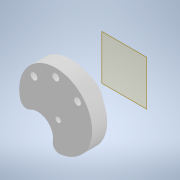
# Autodesk Inventor part: main_wheel_fixator_mirror
Saved by Autodesk Inventor 2022 (Build 260153000, 153)
## iProperties
Created: 2024-09-10
Part Number: main_wheel_fixator_mirror
Material: Типовые
Document SubType Name: Modeling
Designer: Andrey
Density: 1 g/cm^3
Appearance: По умолчанию
Author: Andrey
Autodesk Inventor part; units mm, degrees
ref_plane "YZ Plane" through (0, 0, 0) normal (1, 0, 0) x (0, 1, 0)
ref_plane "XZ Plane" through (0, 0, 0) normal (0, 1, 0) x (-1, 0, 0)
ref_plane "XY Plane" through (0, 0, 0) normal (0, 0, 1) x (1, 0, 0)
ref_plane "РабПлоскость1" through (-130.0323, -33.3842, -9.2947) normal (0, 0, 1) x (1, 0, 0)
sketch "Эскиз1" plane through (0, 0, 0) normal (0, 0, 1) x (1, 0, 0)
  circle A0 centre (0, 0) radius 22.5
  dimension "d0" = 45
  constraints: 1 centre point, 1 coincident
  measures "d0" diameter of A0
extrude "Выдавливание1" add sketch "Эскиз1" against normal up to surface (9.2947 mm away)
sketch "Эскиз2" plane through (0, 0, 0) normal (0, 0, 1) x (1, 0, 0)
  arc A0 (-12.5314, -17.4431) -> (-12.5619, -14.5867) centre (-11.1467, -16) ccw projected
  circle A1 centre (-11.1467, -16) radius 6.5
  circle A2 centre (-11.1467, -16) radius 9.5
  point P0 (0, 0)
  dimension "d3" = 13
  dimension "d4" = 3
  constraints: 2 centre point, 1 coincident
  measures "d3" diameter of A1
  measures "d4" radial gap between concentric circles of A1 A2
extrude "Выдавливание2" cut sketch "Эскиз2" against normal blind 10 contours A1 | A2
fillet "Сопряжение1" radius 4 2 edges at (-3.9122, -22.1573, -4.6474) (-19.4292, -11.347, -4.6474)
sketch "Эскиз3" plane through (0, 0, 0) normal (0, 0, 1) x (1, 0, 0)
  circle A0 centre (0, 0) radius 12.6
  line L0 (0, 0) -> (0, -4)
  line L1 (0, -4) -> (-3.4641, -2)
  line L2 (-3.4641, -2) -> (-3.4641, 2)
  line L3 (-3.4641, 2) -> (0, 4)
  line L4 (0, 4) -> (3.4641, 2)
  line L5 (3.4641, 2) -> (3.4641, -2)
  line L6 (3.4641, -2) -> (0, -4)
  line L7 (-3.9641, -2.2887) -> (0, -4.5774)
  line L8 (0, -4.5774) -> (3.9641, -2.2887)
  line L9 (3.9641, -2.2887) -> (3.9641, 2.2887)
  line L10 (3.9641, 2.2887) -> (0, 4.5774)
  line L11 (0, 4.5774) -> (-3.9641, 2.2887)
  line L12 (-3.9641, 2.2887) -> (-3.9641, -2.2887)
  arc A1 (-21.8671, -5.2989) -> (-15.9551, -7.8067) centre (-17.9796, -4.3569) ccw projected
  arc A2 (-1.795, -17.6717) -> (-15.9551, -7.8067) centre (-11.1467, -16) ccw projected
  arc A3 (-1.795, -17.6717) -> (2.6059, -22.3486) centre (2.1426, -18.3755) ccw projected
  arc A4 (2.6059, -22.3486) -> (-21.8671, -5.2989) centre (0, 0) ccw projected
  point P0 (-10.7899, -6.5067)
  point P1 (-2.3651, -12.376)
  dimension "d8" = 25.2
  dimension "d9" = 4
  dimension "d10" = 0.5
  constraints: 26 end point, 2 coincident, 1 centre point, 1 vertical, 18 other
  measures "d8" diameter of A0
  measures "d9" distance of L0.start L0.end
  measures "d10" distance between parallel lines of L1 L7
extrude "Выдавливание3" add sketch "Эскиз3" along normal blind 7.8 contours A0 A2 picked at (6.8427, 0)
sketch "Эскиз4" plane through (0, 0, 0) normal (0, 0, 1) x (1, 0, 0)
  arc A0 (-2.3651, -12.376) -> (-10.7899, -6.5067) centre (0, 0) ccw projected
  arc A1 (-1.795, -17.6717) -> (-2.3651, -12.376) centre (-11.1467, -16) ccw projected
  arc A2 (-1.795, -17.6717) -> (2.6059, -22.3486) centre (2.1426, -18.3755) ccw projected
  arc A3 (2.6059, -22.3486) -> (-21.8671, -5.2989) centre (0, 0) ccw projected
  arc A4 (-21.8671, -5.2989) -> (-15.9551, -7.8067) centre (-17.9796, -4.3569) ccw projected
  arc A5 (-10.7899, -6.5067) -> (-15.9551, -7.8067) centre (-11.1467, -16) ccw projected
  circle A6 centre (0, 0) radius 12.6
  circle A7 centre (0, 0) radius 14.6
  point P0 (-1.7671, -14.4927)
  point P1 (-12.9827, -6.6791)
  dimension "d13" = 2
  constraints: 2 centre point, 1 coincident, 1 concentric
  measures "d13" radial gap between concentric circles of A6 A7
extrude "Выдавливание4" add sketch "Эскиз4" along normal blind 1 contours A0 A5 A7 A1
fillet "Сопряжение2" radius 2 4 edges at (-2.3651, -12.376, 4.4) (-1.7671, -14.4927, 0.5) (-10.7899, -6.5067, 4.4) (-12.9827, -6.6791, 0.5)
chamfer "Фаска1" distance 0.5 angle 45 7 edges at (8.3458, 11.9795, 1) (-12.8509, -6.1946, 1) (-11.2228, -6.5003, 1) (-10.3052, -6.5373, 1) (-1.3582, -14.2012, 1) (-2.2091, -12.7799, 1) (-2.5618, -11.932, 1)
sketch "Эскиз5" plane through (0, 0, -9.2947) normal (0, 0, -1) x (-0.8205128, 0.5716281, 0)
  circle A0 centre (-6.9744, -14.6412) radius 1.5
  arc A1 (5.5942, -23.7713) -> (7.8344, -23.1299) centre (6.9744, -24.3588) ccw
  arc A2 (5.5942, -23.7713) -> (5.8702, -23.7046) centre (0, 0) ccw
  spline S0 degree 3 poles (7.0407, -25.2882) (6.986, -25.2268) (6.8766, -25.1041) (6.7176, -24.9155) (6.5628, -24.7236) (6.4128, -24.5278) (6.2678, -24.3283) (6.1284, -24.1248) (6.0175, -23.9518) (5.9319, -23.8114) (5.8908, -23.7402) (5.8702, -23.7046) knots 0 0 0 0 0.125 0.250001 0.375002 0.500002 0.625001 0.75 0.874998 0.937499 1 1 1 1
  arc A3 (7.0407, -25.2882) -> (7.5579, -25.1384) centre (0, 0) ccw
  spline S1 degree 3 poles (7.7014, -23.1745) (7.703, -23.2156) (7.7063, -23.2977) (7.709, -23.4621) (7.7076, -23.6676) (7.6985, -23.9141) (7.6826, -24.1602) (7.6603, -24.4058) (7.632, -24.6508) (7.5984, -24.8952) (7.5714, -25.0573) (7.5579, -25.1384) knots 0 0 0 0 0.062501 0.125002 0.25 0.374999 0.499998 0.624998 0.749999 0.875 1 1 1 1
  arc A4 (7.7014, -23.1745) -> (7.8344, -23.1299) centre (0, 0) ccw
  circle A5 centre (0, -19.5) radius 4.5
  line L0 (-92.3726, 48.2814) -> (-109.8668, 39.9786)
  line L1 (13.2101, -45.7656) -> (-109.8668, 39.9786)
  line L2 (13.2101, -45.7656) -> (14.9372, -26.4783)
  arc A6 (18.1683, -19.9728) -> (14.9372, -26.4783) centre (24.8973, -27.3701) ccw
  arc A7 (18.1683, -19.9728) -> (-19.7633, 18.396) centre (0, 0) ccw
  arc A8 (-26.2813, 17.7001) -> (-19.7633, 18.396) centre (-23.4232, 21.8026) ccw
  line L3 (-26.2813, 17.7001) -> (-36.6493, 24.9232)
  arc A9 (-38.2549, 31.2785) -> (-36.6493, 24.9232) centre (-33.7911, 29.0257) ccw
  arc A10 (-38.2549, 31.2785) -> (-87.3896, 53.5664) centre (-62.359, 43.4437) ccw
  arc A11 (-92.3726, 48.2814) -> (-87.3896, 53.5664) centre (-96.6602, 57.3156) ccw
  circle A12 centre (-4.5825, 16.9412) radius 2.1
  circle A13 centre (10.0321, 14.4) radius 2.1
  circle A14 centre (17.4795, 1.5711) radius 2.1
  circle A15 centre (10.0321, 14.4) radius 3.5
  circle A16 centre (-4.5825, 16.9412) radius 3.5
  circle A17 centre (17.4795, 1.5711) radius 3.5
  circle A18 centre (-52.3269, 57.8437) radius 3.5
  circle A19 centre (-44.8794, 45.0149) radius 3.5
  circle A20 centre (-66.9415, 60.3849) radius 3.5
  circle A21 centre (-63.7005, 38.894) radius 1.5
  circle A22 centre (-3.8031, -2.8349) radius 1.5
  circle A23 centre (-39.8968, 9.209) radius 1.5
  point P0 (0, 0)
  dimension "d20" = 4.2
  dimension "d21" = 4.2
  dimension "d22" = 4.2
  constraints: 3 centre point
  measures "d20" diameter of A12
  measures "d21" diameter of A13
  measures "d22" diameter of A14
extrude "Выдавливание5" cut sketch "Эскиз5" against normal blind 7.5 contours A12 | A13 | A14
sketch "Эскиз6" plane through (0, 0, 7.8) normal (0, 0, 1) x (1, 0, 0)
  circle A0 centre (1.5, -4.5) radius 1.5 projected
  circle A1 centre (1.5, -4.5) radius 1.6
  point P0 (0, 0)
  dimension "d25" = 3.2
  constraints: 1 centre point, 1 coincident
  measures "d25" diameter of A1
extrude "Выдавливание6" cut sketch "Эскиз6" against normal blind 20 contours A0 | A1
sketch "Эскиз7" plane through (0, 0, 7.8) normal (0, 0, 1) x (1, 0, 0)
  circle A0 centre (1.5, -4.5) radius 1.5 projected
  circle A1 centre (1.5, -4.5) radius 3.5
  point P0 (0, 0)
  dimension "d28" = 7
  constraints: 1 centre point, 1 coincident
  measures "d28" diameter of A1
extrude "Выдавливание7" cut sketch "Эскиз7" against normal blind 13 contours A0 | A1
ref_plane "РабПлоскость2" through (0, 0, 33.05) normal (0, 0, 1) x (1, 0, 0)
mirror "Зеркальное отражение1" about plane through (0, 0, 33.05) normal (0, 0, 1)
sketch "Эскиз8" plane through (0, 0, -9.2947) normal (0, 0, -1) x (-0.8205128, 0.5716281, 0)
  circle A0 centre (0, 0) radius 41.7428
  constraints: 1 centre point, 1 coincident
extrude "Выдавливание8" cut sketch "Эскиз8" against normal blind 20
